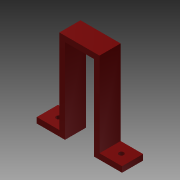
# Autodesk Inventor part: clip
Saved by Autodesk Inventor 2013 (Build 170138000, 138)
## iProperties
Created: 2014-10-25
Part Number: clip
Material: ABS Plastic
Document SubType Name: Modeling
Designer: Masta
Density: 1 g/cm^3
Author: Masta
Autodesk Inventor part; units mm, degrees
ref_plane "YZ Plane" through (0, 0, 0) normal (1, 0, 0) x (0, 1, 0)
ref_plane "XZ Plane" through (0, 0, 0) normal (0, 1, 0) x (-1, 0, 0)
ref_plane "XY Plane" through (0, 0, 0) normal (0, 0, 1) x (1, 0, 0)
sketch "Sketch1" plane through (0, 0, 0) normal (0, 1, 0) x (-1, 0, 0)
  line L0 (0, 0) -> (-10.25, 0)
  line L1 (-10.25, 0) -> (-10.25, -60)
  line L2 (-14.25, 4) -> (0, 4)
  line L3 (0, 4) -> (0, 0)
  line L4 (-10.25, -60) -> (-30.25, -60)
  line L5 (-30.25, -60) -> (-30.25, -56)
  line L6 (-30.25, -56) -> (-14.25, -56)
  line L7 (-14.25, -56) -> (-14.25, 4)
  dimension "d0" = 10.25
  dimension "d1" = 60
  dimension "d3" = 4
  dimension "d4" = 20
  dimension "d5" = 4
  dimension "d6" = 4
  constraints: 16 end point, 4 perpendicular, 3 parallel, 1 horizontal
  measures "d0" distance of L0.start L0.end
  measures "d1" distance of L0.end L1.end
  measures "d3" distance of L2.end L0.start
  measures "d4" distance of L1.end L4.end
  measures "d5" distance of L4.end L5.end
  measures "d6" distance between parallel lines of L1 L7
extrude "Extrusion1" add sketch "Sketch1" along normal blind 15
sketch "Sketch2" plane through (14.25, 0, -56) normal (0, 0, 1) x (1, 0, 0)
  line L0 (0, 15) -> (16, 0) construction
  line L1 (0, 0) -> (16, 15) construction
  point P0 (-14.25, 0)
  point P1 (8, 7.5)
  constraints: 4 end point, 2 midpoint
hole "Hole1" at (22.25, 7.5, -56) direction (0, 0, -1) diameter 3.5 depth 8 tip angle 118
mirror "Mirror1" about plane through (0, 0, 0) normal (-1, 0, 0)
body "Solid1"
